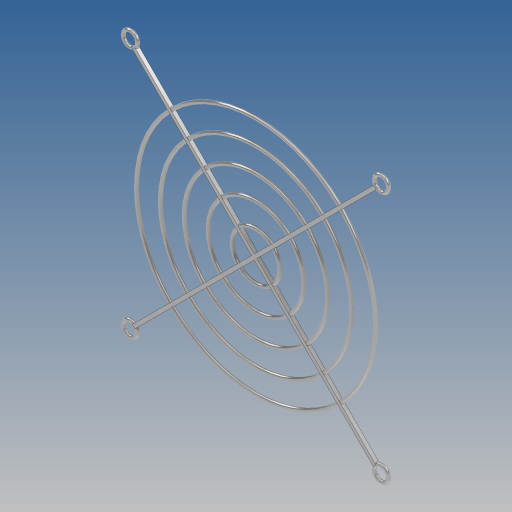
# Autodesk Inventor part: Lüftergitter 1,0
Saved by Autodesk Inventor 2023.3 (Build 273359000, 359)
## iProperties
Created: 2024-01-26
Part Number: Lüftergitter 1,0
Material: Generisch
Document SubType Name: Modeling
Designer: baerchri
Density: 1 g/cm^3
Appearance: Gehont
Author: baerchri
Autodesk Inventor part; units mm, degrees
ref_plane "YZ Plane" through (0, 0, 0) normal (1, 0, 0) x (0, 1, 0)
ref_plane "XZ Plane" through (0, 0, 0) normal (0, 1, 0) x (-1, 0, 0)
ref_plane "XY Plane" through (0, 0, 0) normal (0, 0, 1) x (1, 0, 0)
sketch "Skizze1" plane through (0, 0, 0) normal (0, 0, 1) x (1, 0, 0)
  line L0 (-52.5, -52.5) -> (52.5, -52.5)
  line L1 (52.5, -52.5) -> (52.5, 52.5)
  line L2 (52.5, 52.5) -> (-52.5, 52.5)
  line L3 (-52.5, 52.5) -> (-52.5, -52.5)
  line L4 (-52.5, -52.5) -> (52.5, 52.5) construction
  line L5 (52.5, -52.5) -> (-52.5, 52.5) construction
  circle A0 centre (-52.5, 52.5) radius 2.25
  circle A1 centre (52.5, 52.5) radius 2.25
  circle A2 centre (52.5, -52.5) radius 2.25
  circle A3 centre (-52.5, -52.5) radius 2.25
  circle A4 centre (-52.5, 52.5) radius 3.75
  circle A5 centre (52.5, 52.5) radius 3.75
  circle A6 centre (52.5, -52.5) radius 3.75
  circle A7 centre (-52.5, -52.5) radius 3.75
  line L6 (-52.5, -52.5) -> (52.5, 52.5)
  line L7 (-52.5, 52.5) -> (52.5, -52.5)
  circle A8 centre (0, 0) radius 50.75
  circle A9 centre (0, 0) radius 49.25
  circle A10 centre (0, 0) radius 40.75
  circle A11 centre (0, 0) radius 39.25
  circle A12 centre (0, 0) radius 30.75
  circle A13 centre (0, 0) radius 29.25
  circle A14 centre (0, 0) radius 20.75
  circle A15 centre (0, 0) radius 19.25
  circle A16 centre (0, 0) radius 10.75
  circle A17 centre (0, 0) radius 9.25
  circle A18 centre (0, 0) radius 4.25
  circle A19 centre (0, 0) radius 5.75
  line L8 (-51.4393, 52.5) -> (52.5, -51.4393)
  line L9 (51.4393, -52.5) -> (-52.5, 51.4393)
  line L10 (51.4393, 52.5) -> (-52.5, -51.4393)
  line L11 (-51.4393, -52.5) -> (52.5, 51.4393)
  point P0 (-50.4323, 49.3716)
  point P1 (-36.4121, 35.3514)
  point P2 (-36.4121, -35.3514)
  point P3 (-50.4323, -49.3716)
  point P4 (-49.3716, -50.4323)
  point P5 (-35.3514, -36.4121)
  point P6 (35.3514, -36.4121)
  point P7 (49.3716, -50.4323)
  point P8 (50.4323, -49.3716)
  point P9 (36.4121, -35.3514)
  point P10 (36.4121, 35.3514)
  point P11 (50.4323, 49.3716)
  point P12 (49.3716, 50.4323)
  point P13 (35.3514, 36.4121)
  point P14 (-35.3514, 36.4121)
  point P15 (-49.3716, 50.4323)
  point P16 (3.4884, -2.4277)
  point P17 (3.4884, 2.4277)
  point P18 (7.0495, 5.9889)
  point P19 (7.0495, -5.9889)
  point P20 (8.1132, -7.0525)
  point P21 (8.1132, 7.0525)
  point P22 (14.1318, 13.0711)
  point P23 (14.1318, -13.0711)
  point P24 (15.1932, -14.1325)
  point P25 (15.1932, 14.1325)
  point P26 (21.2064, 20.1457)
  point P27 (21.2064, -20.1457)
  point P28 (22.2674, -21.2067)
  point P29 (22.2674, 21.2067)
  point P30 (28.2792, 27.2185)
  point P31 (28.2792, -27.2185)
  point P32 (29.3401, -28.2794)
  point P33 (29.3401, 28.2794)
  point P34 (35.3513, 34.2906)
  point P35 (35.3513, -34.2906)
  point P36 (34.2906, -35.3513)
  point P37 (-34.2906, -35.3513)
  point P38 (-28.2794, -29.3401)
  point P39 (28.2794, -29.3401)
  point P40 (27.2185, -28.2792)
  point P41 (-27.2185, -28.2792)
  point P42 (-21.2067, -22.2674)
  point P43 (21.2067, -22.2674)
  point P44 (20.1457, -21.2064)
  point P45 (-20.1457, -21.2064)
  point P46 (-14.1325, -15.1932)
  point P47 (14.1325, -15.1932)
  point P48 (13.0711, -14.1318)
  point P49 (-13.0711, -14.1318)
  point P50 (-7.0525, -8.1132)
  point P51 (7.0525, -8.1132)
  point P52 (5.9889, -7.0495)
  point P53 (-5.9889, -7.0495)
  point P54 (-2.4277, -3.4884)
  point P55 (2.4277, -3.4884)
  point P56 (3.5008, -4.5615)
  point P57 (-3.5008, -4.5615)
  point P58 (0, -1.0607)
  point P59 (-29.3401, 28.2794)
  point P60 (-29.3401, -28.2794)
  point P61 (-35.3513, -34.2906)
  point P62 (-35.3513, 34.2906)
  point P63 (-4.5615, 3.5008)
  point P64 (-1.0607, 0)
  point P65 (-4.5615, -3.5008)
  point P66 (-3.5008, 4.5615)
  point P67 (3.5008, 4.5615)
  point P68 (0, 1.0607)
  point P69 (-22.2674, 21.2067)
  point P70 (-22.2674, -21.2067)
  point P71 (-28.2792, -27.2185)
  point P72 (-28.2792, 27.2185)
  point P73 (-28.2794, 29.3401)
  point P74 (-34.2906, 35.3513)
  point P75 (34.2906, 35.3513)
  point P76 (28.2794, 29.3401)
  point P77 (-15.1932, 14.1325)
  point P78 (-15.1932, -14.1325)
  point P79 (-21.2064, -20.1457)
  point P80 (-21.2064, 20.1457)
  point P81 (-21.2067, 22.2674)
  point P82 (-27.2185, 28.2792)
  point P83 (27.2185, 28.2792)
  point P84 (21.2067, 22.2674)
  point P85 (-8.1132, 7.0525)
  point P86 (-8.1132, -7.0525)
  point P87 (-14.1318, -13.0711)
  point P88 (-14.1318, 13.0711)
  point P89 (-14.1325, 15.1932)
  point P90 (-20.1457, 21.2064)
  point P91 (20.1457, 21.2064)
  point P92 (14.1325, 15.1932)
  point P93 (-3.4884, 2.4277)
  point P94 (-3.4884, -2.4277)
  point P95 (-7.0495, -5.9889)
  point P96 (-7.0495, 5.9889)
  point P97 (-7.0525, 8.1132)
  point P98 (-13.0711, 14.1318)
  point P99 (13.0711, 14.1318)
  point P100 (7.0525, 8.1132)
  point P101 (-5.9889, 7.0495)
  point P102 (5.9889, 7.0495)
  point P103 (2.4277, 3.4884)
  point P104 (-2.4277, 3.4884)
  point P105 (4.5615, -3.5008)
  point P106 (1.0607, 0)
  point P107 (4.5615, 3.5008)
  dimension "d23" = 1.5
  dimension "d27" = 1.5
  dimension "d0" = 105
  dimension "d1" = 105
  dimension "d2" = 4.5
  dimension "d3" = 4.5
  dimension "d4" = 4.5
  dimension "d5" = 4.5
  dimension "d6" = 7.5
  dimension "d7" = 7.5
  dimension "d8" = 7.5
  dimension "d9" = 7.5
  dimension "d10" = 101.5
  dimension "d11" = 98.5
  dimension "d12" = 81.5
  dimension "d13" = 78.5
  dimension "d14" = 61.5
  dimension "d15" = 58.5
  dimension "d16" = 41.5
  dimension "d17" = 38.5
  dimension "d18" = 21.5
  dimension "d19" = 18.5
  dimension "d20" = 8.5
  dimension "d21" = 11.5
  dimension "d24" = 0.75
  dimension "d28" = 0.75
  constraints: 20 centre point, 20 coincident, 16 end point, 8 point on line, 2 collinear, 2 midpoint, 2 parallel, 1 horizontal, 1 perpendicular, 14 other
  measures "d0" distance of L2.end L1.end
  measures "d1" distance of L1.end L0.end
  measures "d2" diameter of A0
  measures "d3" diameter of A1
  measures "d4" diameter of A2
  measures "d5" diameter of A3
  measures "d6" diameter of A4
  measures "d7" diameter of A5
  measures "d8" diameter of A6
  measures "d9" diameter of A7
  measures "d10" diameter of A8
  measures "d11" diameter of A9
  measures "d12" diameter of A10
  measures "d13" diameter of A11
  measures "d14" diameter of A12
  measures "d15" diameter of A13
  measures "d16" diameter of A14
  measures "d17" diameter of A15
  measures "d18" diameter of A16
  measures "d19" diameter of A17
  measures "d20" diameter of A18
  measures "d21" diameter of A19
extrude "Extrusion1" add sketch "Skizze1" along normal blind 1.5 contours L6 A7 L11 A3 | A3 L10 A7 L6 | A3 L11 A7 L0 | L0 A7 L3 A3 | L3 A7 L10 A3 | L6 A8 L11 A7 | A7 L10 A8 L6 | A8 L10 A9 L6 | L6 A9 L11 A8 | A6 L9 A2 L0 | L0 A2 L1 A6 | L11 A9 L9 A8 | A4 L2 A0 L3 | L3 A0 L9 A4 | A8 L9 A9 L10 | A9 L10 A10 L6 | L6 A10 L11 A9 | L9 A8 L7 A6 | A6 L7 A2 L9 | L9 A9 L7 A8 | A4 L8 A0 L2 | L9 A0 L7 A4 | A4 L7 A8 L9 | A8 L7 A9 L9 | A10 L10 A11 L6 | L6 A11 L11 A10 | L7 A8 L8 A6 | A6 L8 A2 L7 | L1 A2 L8 A6 | L7 A9 L8 A8 | L9 A10 L7 A9 | L11 A11 L9 A10 | A5 L1 A1 L2 | L2 A1 L10 A5 | L8 A8 L7 A4 | A4 L7 A0 L8 | A8 L8 A9 L7 | A9 L7 A10 L9 | A10 L9 A11 L10 | A11 L10 A12 L6 | L6 A12 L11 A11 | A5 L11 A1 L1 | L7 A10 L8 A9 | L8 A9 L11 A8 | L9 A11 L7 A10 | L10 A1 L6 A5 | A5 L6 A8 L10 | A8 L10 A9 L8 | A9 L8 A10 L7 | A10 L7 A11 L9 | A12 L10 A13 L6 | L6 A13 L11 A12 | L11 A8 L6 A5 | A5 L6 A1 L11 | L7 A11 L8 A10 | L9 A12 L7 A11 | L11 A13 L9 A12 | A8 L6 A9 L10 | A10 L8 A11 L7 | A11 L7 A12 L9 | A12 L9 A13 L10 | A13 L10 A14 L6 | L6 A14 L11 A13 | L11 A9 L6 A8 | L7 A12 L8 A11 | L8 A11 L11 A10 | L9 A13 L7 A12 | A9 L6 A10 L10 | A10 L10 A11 L8 | A11 L8 A12 L7 | A12 L7 A13 L9 | A14 L10 A15 L6 | L6 A15 L11 A14 | L11 A10 L6 A9 | L7 A13 L8 A12 | L9 A14 L7 A13 | L11 A15 L9 A14 | A10 L6 A11 L10 | A12 L8 A13 L7 | A13 L7 A14 L9 | A14 L9 A15 L10 | A15 L10 A16 L6 | L6 A16 L11 A15 | L11 A11 L6 A10 | L7 A14 L8 A13 | L8 A13 L11 A12 | L9 A15 L7 A14 | A11 L6 A12 L10 | A12 L10 A13 L8 | A13 L8 A14 L7 | A14 L7 A15 L9 | A16 L10 A17 L6 | L6 A17 L11 A16 | L11 A12 L6 A11 | L7 A15 L8 A14 | L9 A16 L7 A15 | L11 A17 L9 A16 | A12 L6 A13 L10 | A14 L8 A15 L7 | A15 L7 A16 L9 | A16 L9 A17 L10 | A17 L10 A19 L6 | L6 A19 L11 A17 | L11 A13 L6 A12 | L7 A16 L8 A15 | L8 A15 L11 A14 | L9 A17 L7 A16 | A13 L6 A14 L10 | A14 L10 A15 L8 | A15 L8 A16 L7 | A16 L7 A17 L9 | A19 L10 A18 L6 | L6 A18 L11 A19 | L11 A14 L6 A13 | L7 A17 L8 A16 | L9 A19 L7 A17 | A14 L6 A15 L10 | A16 L8 A17 L7 | A17 L7 A19 L9 | A18 L10 L9 L6 | L6 L9 L11 A18 | L11 A15 L6 A14 | L7 A19 L8 A17 | L8 A17 L11 A16 | L9 A18 L7 A19 | A15 L6 A16 L10 | A16 L10 A17 L8 | A17 L8 A19 L7 | A19 L7 A18 L9 | L9 L10 L7 L6 | L6 L7 L11 L9 | L11 A16 L6 A15 | L7 A18 L8 A19 | L9 L11 L7 A18 | A16 L6 A17 L10 | A19 L8 A18 L7 | A18 L7 L10 L9 | L7 L10 L8 L6 | L6 L8 L11 L7 | L11 A17 L6 A16 | L7 L11 L8 A18 | A17 L6 A19 L10 | A18 L8 L10 L7 | L8 L10 A18 L6 | L6 A18 L11 L8 | L11 A19 L6 A17 | A19 L6 A18 L10 | L6 A19 L11 A18
fillet "Rundung1" radius 0.75 80 edges at (-49.25, 0, 1.5) (-50.75, 0, 1.5) (-50.75, 0, 0) (-49.25, 0, 0) (-40.75, 0, 1.5) (-39.25, 0, 1.5) (-30.75, 0, 1.5) (-29.25, 0, 1.5) (-20.75, 0, 1.5) (-19.25, 0, 1.5) (-10.75, 0, 1.5) (-9.25, 0, 1.5) (0, -9.25, 1.5) (0, -10.75, 1.5) (0, -19.25, 1.5) (0, -20.75, 1.5) (0, -29.25, 1.5) (0, -30.75, 1.5) (0, -39.25, 1.5) (0, -40.75, 1.5) (0, -49.25, 1.5) (0, -50.75, 1.5) (10.75, 0, 1.5) (9.25, 0, 1.5) (19.25, 0, 1.5) (20.75, 0, 1.5) (29.25, 0, 1.5) (30.75, 0, 1.5) (39.25, 0, 1.5) (40.75, 0, 1.5) (49.25, 0, 1.5) (50.75, 0, 1.5) (0, 10.75, 1.5) (0, 9.25, 1.5) (0, 19.25, 1.5) (0, 20.75, 1.5) (0, 29.25, 1.5) (0, 30.75, 1.5) (0, 39.25, 1.5) (0, 40.75, 1.5) (0, 49.25, 1.5) (0, 50.75, 1.5) (0, 50.75, 0) (0, 49.25, 0) (0, 40.75, 0) (0, 39.25, 0) (0, 30.75, 0) (0, 29.25, 0) (0, 20.75, 0) (0, 19.25, 0) (29.25, 0, 0) (30.75, 0, 0) (39.25, 0, 0) (40.75, 0, 0) (49.25, 0, 0) (50.75, 0, 0) (20.75, 0, 0) (19.25, 0, 0) (10.75, 0, 0) (9.25, 0, 0) (0, 10.75, 0) (0, 9.25, 0) (-9.25, 0, 0) (-10.75, 0, 0) (0, -10.75, 0) (0, -9.25, 0) (0, -19.25, 0) (0, -20.75, 0) (0, -29.25, 0) (0, -30.75, 0) (0, -39.25, 0) (0, -40.75, 0) (0, -49.25, 0) (0, -50.75, 0) (-19.25, 0, 0) (-20.75, 0, 0) (-29.25, 0, 0) (-30.75, 0, 0) (-39.25, 0, 0) (-40.75, 0, 0)
fillet "Rundung2" radius 0.75 16 edges at (50.25, -52.5, 0) (55.1517, -55.1517, 1.5) (55.1517, -55.1517, 0) (50.25, -52.5, 1.5) (-54.75, -52.5, 0) (-54.75, -52.5, 1.5) (-55.1517, -55.1517, 1.5) (-55.1517, -55.1517, 0) (-54.75, 52.5, 1.5) (-54.75, 52.5, 0) (-55.1517, 55.1517, 1.5) (-55.1517, 55.1517, 0) (50.25, 52.5, 1.5) (55.1517, 55.1517, 1.5) (50.25, 52.5, 0) (55.1517, 55.1517, 0)
equation "\"d27\" = d23"
equation "\"d3\" = d2"
equation "\"d4\" = d2"
equation "\"d5\" = d2"
equation "\"d7\" = d6"
equation "\"d8\" = d6"
equation "\"d9\" = d6"
equation "\"d24\" = 0.5 * d23"
equation "\"d28\" = d24"
